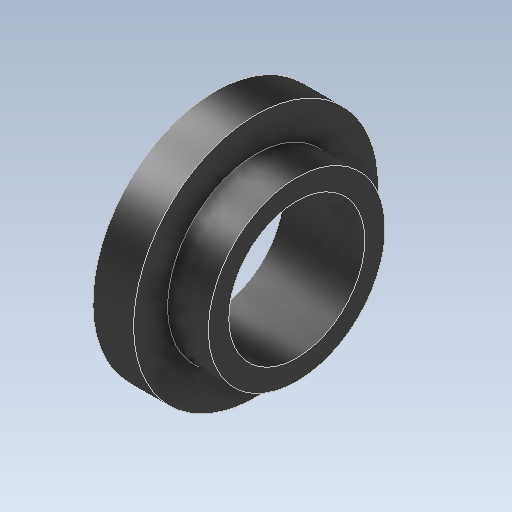
# Autodesk Inventor part: Peça16
Saved by Autodesk Inventor 2021 (Build 250183000, 183)
## iProperties
Category: 41
Created: 2021-07-18
Part Number: Peça16
Material: Aço
Document SubType Name: Modeling
Designer: Giovanni
Density: 7.85 g/cm^3
Appearance: Brilhosa - Preta
User Status: 3:1
Author: Giovanni
Keywords: 15
Autodesk Inventor part; units mm, degrees
ref_plane "YZ Plane" through (0, 0, 0) normal (1, 0, 0) x (0, 1, 0)
ref_plane "XZ Plane" through (0, 0, 0) normal (0, 1, 0) x (-1, 0, 0)
ref_plane "XY Plane" through (0, 0, 0) normal (0, 0, 1) x (1, 0, 0)
sketch "Esboço1" plane through (0, 0, 0) normal (0, 0, 1) x (1, 0, 0)
  line L0 (0, 5) -> (6, 5)
  line L1 (6, 5) -> (6, 6.5)
  line L2 (6, 6.5) -> (3, 6.5)
  line L3 (3, 6.5) -> (3, 9)
  line L4 (3, 9) -> (0, 9)
  line L5 (0, 9) -> (0, 5)
  line L6 (-1.2, 0) -> (7.2, 0) projected
  point P0 (0, 0)
  dimension "d0" = 5
  dimension "d1" = 6
  dimension "d2" = 6.5
  dimension "d3" = 9
  dimension "d4" = 3
  constraints: 12 end point, 5 perpendicular, 1 horizontal, 1 vertical alignment
  measures "d0" distance from line of L0 point (0, 0)
  measures "d1" distance of L0.start L0.end
  measures "d2" distance from line of L2 point (0, 0)
  measures "d3" distance from line of L4 point (0, 0)
  measures "d4" distance of L3.end L4.end
revolve "Revolução1" add sketch "Esboço1" angle 360 about axis through (-10, 0, 0) along (-1, 0, 0)
